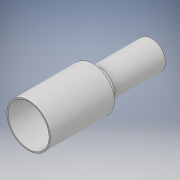
# Autodesk Inventor part: 5mm to 8mm holder
Saved by Autodesk Inventor 2018 (Build 220112000, 112)
## iProperties
Created: 2017-11-24
Part Number: 5mm to 8mm holder
Material: Generic
Document SubType Name: Modeling
Designer: g
Density: 1 g/cm^3
Appearance: Default
Author: g
Autodesk Inventor part; units mm, degrees
ref_plane "YZ Plane" through (0, 0, 0) normal (1, 0, 0) x (0, 1, 0)
ref_plane "XZ Plane" through (0, 0, 0) normal (0, 1, 0) x (-1, 0, 0)
ref_plane "XY Plane" through (0, 0, 0) normal (0, 0, 1) x (1, 0, 0)
ref_plane "Work Plane3" through (0, 10, 0) normal (0, 1, 0) x (1, 0, 0)
sketch "Sketch2" plane through (0, 10, 0) normal (0, 1, 0) x (1, 0, 0)
  circle A0 centre (0, 0) radius 4
  circle A1 centre (0, 0) radius 4.25
  dimension "d4" = 8
  dimension "d5" = 0.25
  constraints: 2 centre point, 1 coincident
  measures "d4" diameter of A0
  measures "d5" radial gap between concentric circles of A0 A1
extrude "Extrusion2" add sketch "Sketch2" along normal blind 15
extrude "Extrusion3" cut sketch "Sketch2" along normal blind 2.5
ref_plane "Work Plane1" through (0, 11.25, 0) normal (0, 1, 0) x (1, 0, 0)
ref_plane "Work Plane2" through (0, 26.5, 0) normal (0, 1, 0) x (1, 0, 0)
sketch "Sketch6" plane through (0, 26.5, 0) normal (0, 1, 0) x (1, 0, 0)
  circle A0 centre (0, 0) radius 2.75
  dimension "d17" = 5.5
  constraints: 1 centre point, 1 coincident
  measures "d17" diameter of A0
loft "Loft1" add profiles "Sketch6" section 1 edges at (-4.25, 25, 0)
sketch "Sketch7" plane through (0, 26.5, 0) normal (0, 1, 0) x (1, 0, 0)
  circle A0 centre (0, 0) radius 2.5
  dimension "d22" = 5
  constraints: 1 centre point, 1 coincident
  measures "d22" diameter of A0
extrude "Extrusion4" cut sketch "Sketch7" against normal blind 2.5
sketch "Sketch8" plane through (0, 26.5, 0) normal (0, 1, 0) x (1, 0, 0)
  circle A0 centre (0, 0) radius 2.75
  circle A1 centre (0, 0) radius 2.5
  dimension "d25" = 5.5
  dimension "d26" = 0.25
  constraints: 2 centre point, 1 coincident
  measures "d25" diameter of A0
  measures "d26" radial gap between concentric circles of A0 A1
extrude "Extrusion5" add sketch "Sketch8" along normal blind 10
body "Solid1"
